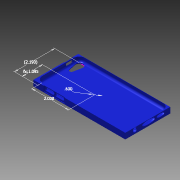
# Autodesk Inventor part: ipodcasev4
Saved by Autodesk Inventor 2014 SP2 (Build 180246200, 246)
## iProperties
Created: 2013-11-12
Part Number: ipodcasev4
Material: Generic
Document SubType Name: Modeling
Designer: jared.hale
Density: 1 g/cm^3
Appearance: Blue - Wall Paint - Glossy
Author: jared.hale
Autodesk Inventor part; units mm, degrees
ref_plane "YZ Plane" through (0, 0, 0) normal (1, 0, 0) x (0, 1, 0)
ref_plane "XZ Plane" through (0, 0, 0) normal (0, 1, 0) x (-1, 0, 0)
ref_plane "XY Plane" through (0, 0, 0) normal (0, 0, 1) x (1, 0, 0)
sketch "Sketch1" plane through (0, 0, 0) normal (0, 1, 0) x (-1, 0, 0)
  line L0 (-133.35, 69.85) -> (0, 69.85)
  line L1 (0, 69.85) -> (0, 0)
  line L2 (0, 0) -> (-133.35, 0)
  line L3 (-133.35, 0) -> (-133.35, 69.85)
  dimension "d0" = 133.35
  dimension "d2" = 69.85
  constraints: 8 end point, 2 parallel, 1 horizontal, 1 perpendicular
  measures "d0" distance between parallel lines of L1 L3
  measures "d2" distance between parallel lines of L2 L0
extrude "Extrusion1" add sketch "Sketch1" along normal blind 25.4
sketch "Sketch2" plane through (0, 25.4, 0) normal (0, 1, 0) x (1, 0, 0)
  line L0 (0, 0) -> (0, -69.85) projected
  line L1 (133.35, 0) -> (0, 0) projected
  line L2 (12.7, -5.08) -> (121.285, -5.08)
  line L3 (128.905, -12.7) -> (128.905, -56.388)
  line L4 (121.285, -64.008) -> (12.7, -64.008)
  line L5 (5.08, -56.388) -> (5.08, -12.7)
  arc A0 (12.7, -5.08) -> (5.08, -12.7) centre (12.7, -12.7) ccw
  arc A1 (5.08, -56.388) -> (12.7, -64.008) centre (12.7, -56.388) ccw
  arc A2 (121.285, -64.008) -> (128.905, -56.388) centre (121.285, -56.388) ccw
  arc A3 (128.905, -12.7) -> (121.285, -5.08) centre (121.285, -12.7) ccw
  dimension "d5" = 58.928
  dimension "d7" = 123.825
  dimension "d8" = 5.08
  dimension "d9" = 5.08
  dimension "d10" = 7.62
  constraints: 8 end point, 8 point on circle, 8 tangent, 4 centre point, 3 equal radius, 2 parallel, 1 horizontal, 1 perpendicular
  measures "d5" distance between parallel lines of L4 L2
  measures "d7" distance between parallel lines of L3 L5
  measures "d8" distance between parallel lines of L2 L1
  measures "d9" distance between parallel lines of L0 L5
  measures "d10" radius of A0
extrude "Extrusion2" cut sketch "Sketch2" against normal blind 6.4008
fillet "Fillet1" radius 3.175 8 edges at (126.6732, 18.9992, 7.3118) (128.905, 18.9992, 34.544) (126.6732, 18.9992, 61.7762) (66.9925, 18.9992, 64.008) (7.3118, 18.9992, 61.7762) (5.08, 18.9992, 34.544) (7.3118, 18.9992, 7.3118) (66.9925, 18.9992, 5.08)
sketch "Sketch3" plane through (5.08, 25.4, 56.388) normal (1, 0, 0) x (0, 0, -1)
  line L0 (43.688, 0) -> (43.688, -3.2258) projected
  line L1 (0, 0) -> (43.688, 0) projected
  line L2 (34.163, -1.397) -> (41.402, -1.397)
  line L3 (42.672, -2.667) -> (42.672, -3.175)
  line L4 (41.402, -4.445) -> (34.163, -4.445)
  line L5 (32.893, -3.175) -> (32.893, -2.667)
  arc A0 (42.672, -2.667) -> (41.402, -1.397) centre (41.402, -2.667) ccw
  arc A1 (41.402, -4.445) -> (42.672, -3.175) centre (41.402, -3.175) ccw
  arc A2 (32.893, -3.175) -> (34.163, -4.445) centre (34.163, -3.175) ccw
  arc A3 (34.163, -1.397) -> (32.893, -2.667) centre (34.163, -2.667) ccw
  point P0 (56.388, -25.4)
  dimension "d14" = 1.016
  dimension "d15" = 9.779
  dimension "d16" = 1.397
  dimension "d17" = 3.048
  dimension "d18" = 1.27
  constraints: 8 end point, 8 point on circle, 8 tangent, 4 centre point, 3 equal radius, 2 parallel, 1 horizontal, 1 perpendicular
  measures "d14" distance between parallel lines of L3 L0
  measures "d15" distance between parallel lines of L5 L3
  measures "d16" distance between parallel lines of L2 L1
  measures "d17" distance between parallel lines of L4 L2
  measures "d18" radius of A0
extrude "Extrusion3" cut sketch "Sketch3" along normal mid plane 50.8
sketch "Sketch4" plane through (121.285, 25.4, 64.008) normal (0, 0, -1) x (-1, 0, 0)
  line L0 (0, 0) -> (108.585, 0) projected
  line L1 (77.851, -4.953) -> (100.711, -4.953)
  line L2 (101.981, -3.683) -> (101.981, -2.54)
  line L3 (100.711, -1.27) -> (77.851, -1.27)
  line L4 (76.581, -2.54) -> (76.581, -3.683)
  arc A0 (101.981, -2.54) -> (100.711, -1.27) centre (100.711, -2.54) ccw
  arc A1 (100.711, -4.953) -> (101.981, -3.683) centre (100.711, -3.683) ccw
  arc A2 (77.851, -1.27) -> (76.581, -2.54) centre (77.851, -2.54) ccw
  arc A3 (76.581, -3.683) -> (77.851, -4.953) centre (77.851, -3.683) ccw
  point P0 (108.585, -3.2258)
  point P1 (121.285, -25.4)
  point P2 (116.205, -3.2258)
  dimension "d37" = 7.62
  dimension "d38" = 14.224
  dimension "d39" = 25.4
  dimension "d40" = 3.683
  dimension "d41" = 3.2258
  dimension "d42" = 1.27
  dimension "d43" = 1.27
  constraints: 8 end point, 8 point on circle, 8 tangent, 4 centre point, 3 equal radius, 2 parallel, 1 horizontal, 1 perpendicular
  measures "d37" distance of point (108.585, -3.226) point (116.205, -3.226)
  measures "d38" distance from line of point (116.205, -3.226) L2
  measures "d39" distance between parallel lines of L4 L2
  measures "d40" distance between parallel lines of L1 L3
  measures "d41" distance from line of point (116.205, -3.226) L0
  measures "d42" distance between parallel lines of L3 L0
  measures "d43" radius of A0
sketch "Sketch5" plane through (128.905, 25.4, 12.7) normal (-1, 0, 0) x (0, 0, 1)
  line L0 (43.688, -3.2258) -> (0, -3.2258) projected
  line L1 (0, 0) -> (43.688, 0) projected
  ellipse E0 centre (21.7805, -3.175) end of major axis (30.6705, -3.175) minor radius 2.54
  point P0 (-12.7, -25.4)
  dimension "d21" = 8.89
  dimension "d23" = 2.54
  dimension "d26" = 3.175
  constraints: 1 horizontal, 2 other
  measures "d26" distance from line of point (21.78, -3.175) L1
extrude "Extrusion4" cut sketch "Sketch5" along normal mid plane 50.8
sketch "Sketch6" plane through (128.905, 25.4, 12.7) normal (-1, 0, 0) x (0, 0, 1)
  ellipse E0 centre (21.7805, -3.175) end of major axis (12.8905, -3.175) minor radius 2.54 (30.6687, -3.2258) -> (12.8923, -3.2258) ccw projected
  line L0 (12.8923, -3.2258) -> (0, -3.2258) projected
  circle A0 centre (40.7035, -3.175) radius 2.794
  ellipse E1 centre (5.2705, -3.175) end of major axis (10.668, -3.175) minor radius 1.905
  point P0 (-12.7, -25.4)
  dimension "d35" = 5.3975
  dimension "d36" = 1.905
  dimension "d29" = 5.588
  dimension "d31" = 18.923
  dimension "d34" = 16.51
  constraints: 1 centre point, 1 horizontal, 3 other
  measures "d29" diameter of A0
  measures "d31" distance of point (21.78, -3.175) A0.centre
  measures "d34" distance of point (5.27, -3.175) point (21.78, -3.175)
extrude "Extrusion5" cut sketch "Sketch6" along normal mid plane 10.16
extrude "Extrusion6" cut sketch "Sketch4" along normal mid plane 50.8
sketch "Sketch7" plane through (0, 18.9992, 0) normal (0, 1, 0) x (1, 0, 0)
  line L0 (12.7, -8.255) -> (121.285, -8.255) projected
  line L1 (8.255, -56.388) -> (8.255, -12.7) projected
  arc A0 (16.7866, -12.9365) -> (7.3434, -12.9365) centre (12.065, -11.938) ccw
  arc A1 (9.58, -23.5125) -> (14.55, -23.5125) centre (12.065, -22.987) ccw
  line L2 (7.3434, -12.9365) -> (9.58, -23.5125)
  line L3 (16.7866, -12.9365) -> (14.55, -23.5125)
  point P0 (0, 0)
  point P1 (5.08, -5.08)
  dimension "d46" = 11.049
  dimension "d48" = 0
  dimension "d49" = 9.652
  dimension "d50" = 5.08
  dimension "d51" = 3.175
  dimension "d52" = 3.175
  dimension "d53" = 6.858
  dimension "d54" = 6.985
  constraints: 4 end point, 4 point on circle, 4 tangent, 2 centre point
  measures "d46" distance of A1.centre A0.centre
  measures "d48" horizontal distance of A0.centre A1.centre
  measures "d49" diameter of A0
  measures "d50" diameter of A1
  measures "d51" distance from line of point (5.08, -5.08) L0
  measures "d52" distance from line of point (5.08, -5.08) L1
  measures "d53" vertical distance of A0.centre point (5.08, -5.08)
  measures "d54" horizontal distance of A0.centre point (5.08, -5.08)
extrude "Extrusion7" cut sketch "Sketch7" along normal mid plane 50.8
ref_plane "Work Plane1" through (0, 0, 34.925) normal (0, 0, 1) x (1, 0, 0)
fillet "Fillet2" [suppressed]
sketch "Sketch10" plane through (0, 0, 34.925) normal (0, 0, 1) x (1, 0, 0)
  line L0 (15.1836, 18.9992) -> (121.285, 18.9992) projected
  line L1 (5.08, 24.13) -> (5.7032, 25.2095) projected
  line L2 (128.905, 24.13) -> (128.2818, 25.2095) projected
  line L3 (3.556, 25.8521) -> (3.556, 17.4752)
  line L4 (3.556, 17.4752) -> (130.429, 17.4752)
  line L5 (130.429, 17.4752) -> (130.429, 25.8521)
  line L6 (3.556, 25.8521) -> (-3.1756, 25.6598)
  line L7 (-3.1756, 25.6598) -> (-4.2851, -9.2303)
  line L8 (-4.2851, -9.2303) -> (140.2506, -12.8123)
  line L9 (140.2506, -12.8123) -> (141.3589, 31.9078)
  line L10 (141.3589, 31.9078) -> (130.429, 25.8521)
  point P0 (0, 0)
  dimension "d62" = 1.524
  dimension "d63" = 1.524
  dimension "d65" = 1.524
  constraints: 16 end point, 1 parallel, 1 perpendicular
  measures "d62" distance from line of L3 L1.start
  measures "d63" distance from line of L5 L2.start
  measures "d65" distance between parallel lines of L4 L0
extrude "Extrusion8" cut sketch "Sketch10" along normal mid plane 127
ref_plane "Work Plane2" through (66.9925, 22.1742, 43.3687) normal (-1, 0, 0) x (0, 0, 1)
sketch "Sketch11" plane through (66.9925, 22.1742, 43.3687) normal (-1, 0, 0) x (0, 0, 1)
  arc A0 (-38.2887, 0) -> (-35.1137, -3.175) centre (-35.1137, 0) ccw projected
  line L0 (-38.2887, 3.2258) -> (-38.2887, 0) projected
  line L1 (-37.019, 1.9558) -> (-36.3957, 3.0353) projected
  line L2 (-35.1137, -3.175) -> (-30.6687, -3.175) projected
  line L3 (-30.6687, -3.175) -> (13.0193, -3.175) projected
  line L4 (21.909, 1.9558) -> (21.2858, 3.0353) projected
  line L5 (20.6393, 3.2258) -> (20.6393, 0) projected
  arc A1 (17.4643, -3.175) -> (20.6393, 0) centre (17.4643, 0) ccw projected
  line L6 (23.433, 3.4455) -> (23.433, -4.699)
  line L7 (23.433, -4.699) -> (-38.543, -4.699)
  line L8 (-38.543, -4.699) -> (-38.543, 3.4455)
  line L9 (-38.543, 3.4455) -> (-45.2909, 4.3376)
  line L10 (-45.2909, 4.3376) -> (-44.8539, -8.6551)
  line L11 (-44.8539, -8.6551) -> (36.1582, -8.6551)
  line L12 (36.1582, -8.6551) -> (31.3237, 8.6218)
  line L13 (31.3237, 8.6218) -> (23.433, 3.4455)
  point P0 (-43.3687, -22.1742)
  point P1 (9.795, -3.175)
  dimension "d68" = 1.524
  dimension "d69" = 1.524
  dimension "d70" = 1.524
  constraints: 16 end point, 1 parallel, 1 perpendicular, 2 other
  measures "d68" distance from line of L8 L1.start
  measures "d69" distance from line of L6 L4.start
  measures "d70" distance between parallel lines of L7 L3
extrude "Extrusion9" cut sketch "Sketch11" along normal mid plane 152.4
sketch "Sketch12" plane through (20.574, 24.13, 66.8017) normal (0, 0, 1) x (1, 0, 0)
  line L0 (22.86, 0) -> (0, 0) projected
  line L1 (-16.764, 1.27) -> (-16.764, -3.4798) projected
  line L2 (10.4775, 0) -> (10.4775, -3.683)
  line L3 (10.4775, -3.683) -> (12.3825, -3.683)
  line L4 (12.3825, -3.683) -> (12.3825, 0)
  line L5 (22.86, -3.683) -> (0, -3.683) projected
  point P0 (-20.574, -24.13)
  point P1 (-16.764, 0.635)
  point P2 (-1.27, -2.413)
  point P3 (24.13, -2.413)
  dimension "d82" = 1.905
  dimension "d85" = 0
  dimension "d91" = 25.4
  dimension "d92" = 11.7475
  constraints: 6 end point, 2 perpendicular, 2 point on line, 1 parallel
  measures "d82" distance between parallel lines of L4 L2
  measures "d85" distance between parallel lines of L5 L3
  measures "d91" distance of point (24.13, -2.413) point (-1.27, -2.413)
  measures "d92" distance from line of point (-1.27, -2.413) L2
extrude "Extrusion10" add sketch "Sketch12" against normal blind 2.54
fillet "Fillet10" radius 1.27 4 edges at (32.9565, 20.447, 65.5317) (32.9565, 24.13, 65.5317) (31.0515, 24.13, 65.5317) (31.0515, 20.447, 65.5317)
chamfer "Chamfer3" distance 0.762 angle 45 4 edges at (12.065, 17.4752, 7.112) (15.6683, 17.4752, 18.2245) (12.065, 17.4752, 25.527) (8.4617, 17.4752, 18.2245)
ref_plane "Work Plane3" through (13.716, 17.4752, 62.357) normal (0, -1, 0) x (1, 0, 0)
sketch "Sketch14" plane through (13.716, 17.4752, 62.357) normal (0, -1, 0) x (1, 0, 0)
  line L0 (113.538, -55.626) -> (-6.985, -55.626) projected
  line L1 (-6.985, 0) -> (113.538, 0) projected
  circle A0 centre (42.164, -27.813) radius 7.62
  line L2 (-8.636, -38.863) -> (-8.636, -5.969) projected
  point P0 (0.4971, -55.499)
  point P1 (106.553, -55.626)
  point P2 (106.553, 0)
  point P3 (0, 0)
  point P4 (-13.716, -62.357)
  point P5 (0.0679, -55.626)
  point P6 (-6.985, -55.626)
  dimension "d103" = 27.813
  dimension "d104" = 55.626
  dimension "d105" = 50.8
  dimension "d106" = 15.24
  constraints: 1 centre point, 1 other
  measures "d103" distance from line of A0.centre L1
  measures "d105" distance from line of A0.centre L2
  measures "d106" diameter of A0
sketch "Sketch17" plane through (0, 25.4, 0) normal (0, 1, 0) x (1, 0, 0)
  line L0 (3.556, -66.8017) -> (130.429, -66.8017) projected
  line L1 (3.556, -4.8257) -> (3.556, -66.8017) projected
  line L2 (5.08, -13.716) -> (3.556, -13.716) projected
  line L3 (3.556, -13.716) -> (5.08, -13.716) projected
  line L4 (5.08, -23.495) -> (3.556, -23.495) projected
  line L5 (5.08, -23.495) -> (3.556, -23.495) projected
  line L6 (4.318, -24.13) -> (4.318, -13.081)
  line L7 (45.72, -66.0397) -> (18.288, -66.0397)
  line L8 (4.318, -24.511) -> (4.318, -24.13)
  line L9 (4.318, -12.7) -> (4.318, -13.157)
  line L10 (4.318, -24.511) -> (3.556, -25.273)
  line L11 (4.318, -24.511) -> (5.471, -24.511) construction
  line L12 (4.318, -12.7) -> (3.7438, -12.1258)
  line L13 (4.318, -12.7) -> (5.2745, -12.7) construction
  line L14 (18.288, -66.0397) -> (17.526, -66.8017)
  line L15 (45.72, -66.0397) -> (46.482, -66.8017)
  arc A0 (12.7, -4.8257) -> (3.556, -13.9697) centre (12.7, -13.9697) ccw projected
  point P0 (3.556, -55.372)
  point P1 (13.716, -65.532)
  point P2 (120.269, -65.532)
  point P3 (3.556, -13.716)
  point P4 (0, 0)
  point P5 (44.704, -66.8017)
  point P6 (32.9565, -66.8017)
  point P7 (31.0515, -66.8017)
  point P8 (19.304, -66.8017)
  point P9 (3.6899, -12.0719)
  dimension "d115" = 0.762
  dimension "d119" = 135
  dimension "d120" = 135
  dimension "d121" = 0.762
  dimension "d122" = 1.016
  dimension "d123" = 1.016
  dimension "d125" = 1.016
  constraints: 20 end point, 3 horizontal, 3 perpendicular, 3 point on line, 2 collinear, 1 point on circle, 3 other
  measures "d115" distance between parallel lines of L6 L1
  measures "d119" angle of L10 L11
  measures "d120" angle of L13 L12
  measures "d122" horizontal distance of point (44.704, -66.802) L7.start
  measures "d123" horizontal distance of point (19.304, -66.802) L7.end
  measures "d125" distance from line of L4 L8.start
extrude "Extrusion13" cut sketch "Sketch17" against normal blind 7.0866 contours L14 L7 L15 L0 | A0 L2 L6 L4 L1 | A0 L12 L9 L6 L2 | L4 L6 L8 L10 L1
fillet "Fillet20" radius 0.5387 4 edges at (18.288, 21.8567, 66.0397) (45.72, 21.8567, 66.0397) (4.318, 21.8567, 12.7) (4.318, 21.8567, 24.511)
fillet "Fillet21" radius 0.254 3 edges at (3.556, 21.8567, 25.273) (17.526, 21.8567, 66.8017) (46.482, 21.8567, 66.8017)
chamfer "Chamfer5" distance 0.762 angle 45 8 edges at (4.318, 20.955, 18.6055) (4.318, 21.327, 23.123) (4.318, 22.479, 23.495) (4.318, 23.631, 23.123) (4.318, 24.003, 18.6055) (4.318, 23.631, 14.088) (4.318, 22.479, 13.716) (4.318, 21.327, 14.088)
fillet "Fillet22" radius 0.762 8 edges at (4.318, 22.479, 12.9541) (4.318, 20.7882, 13.5492) (4.318, 20.1931, 18.6055) (4.318, 20.7882, 23.6618) (4.318, 22.479, 24.2569) (4.318, 24.1698, 23.6618) (4.318, 24.7649, 18.6055) (4.318, 24.1698, 13.5492)
sketch "Sketch18" plane through (32.9565, 20.447, 62.992) normal (1, 0, 0) x (0, 0, -1)
  line L0 (-1.2697, 1.27) -> (-3.0477, 1.27) projected
  arc A0 (-0.9829, 1.27) -> (-0.5051, 0) centre (2.159, 1.7272) ccw projected
  line L1 (-0.5051, 0) -> (0, 0) projected
  line L2 (-1.2697, 2.413) -> (-1.2697, 1.27) projected
  line L3 (-1.016, 3.683) -> (0, 3.683) projected
  line L4 (-1.016, 3.683) -> (-1.016, 2.413) projected
  line L5 (-3.0477, 2.413) -> (-3.0477, 3.683) projected
  line L6 (-3.0477, 3.683) -> (-1.2697, 3.683) projected
  line L7 (-1.2697, 2.413) -> (-3.0477, 2.413) projected
  arc A1 (-0.9829, 1.27) -> (-0.5051, 0) centre (2.159, 1.7272) ccw
  line L8 (-1.016, 3.683) -> (-1.016, 2.413)
  line L9 (-1.016, 2.413) -> (-1.016, 1.27)
  arc A2 (-1.016, 1.8415) -> (-0.9829, 1.27) centre (2.2895, 1.7462) ccw
  line L10 (-1.016, 3.683) -> (0, 3.683)
  line L11 (0, 3.683) -> (0, 0)
  line L12 (0, 0) -> (-0.5051, 0)
  line L13 (-1.2697, 3.683) -> (-1.2697, 2.413) projected
  point P0 (62.992, -20.447)
  constraints: 10 end point, 4 collinear, 4 point on circle, 2 centre point, 1 midpoint, 1 point on line, 1 tangent, 1 vertical, 1 other
extrude "Extrusion14" cut sketch "Sketch18" against normal up to surface (1.905 mm away) contours A2 L9 L4 L3 L11 L1 A0
sketch "Sketch19" plane through (31.0515, 21.717, 66.0397) normal (-1, 0, 0) x (0, 0, 1)
  arc A0 (-0.7951, 0) -> (-0.762, 0.5715) centre (-4.0675, 0.4762) ccw projected
  line L0 (-0.762, 1.143) -> (-0.762, 0.5715) projected
  line L1 (-0.762, 2.159) -> (-0.635, 2.159)
  line L2 (-0.635, 2.159) -> (-0.635, -1.016)
  line L3 (-0.635, -1.016) -> (-2.3942, -1.016)
  arc A1 (-5.2067, -2.7178) -> (-2.0317, 0.4572) centre (-5.2067, 0.4572) ccw projected
  line L4 (-0.762, 2.413) -> (-0.762, 1.143) projected
  line L5 (-0.762, 2.159) -> (-0.762, 0.5715)
  arc A2 (-2.3942, -1.016) -> (-0.762, 0.5715) centre (-2.3068, 0.527) ccw
  point P0 (-66.0397, -21.717)
  point P1 (0, 2.413)
  point P2 (0, -1.27)
  dimension "d140" = 0.254
  dimension "d141" = 0.254
  dimension "d142" = 0.127
  constraints: 8 end point, 2 perpendicular, 2 point on circle, 1 centre point, 1 collinear, 1 parallel, 1 tangent, 2 other
  measures "d140" distance from line of L3 point (0, -1.27)
  measures "d141" distance from line of point (0, 2.413) L1
  measures "d142" distance between parallel lines of L4 L2
extrude "Extrusion15" [suppressed]
fillet "Fillet23" [suppressed]
fillet "Fillet24" radius 0.3175 5 edges at (130.429, 20.32, 17.9689) (130.429, 24.13, 17.9721) (130.429, 19.685, 34.4785) (130.429, 24.765, 34.4823) (130.429, 22.225, 50.6095)
chamfer "Chamfer6" distance 0.381 angle 45 16 edges at (31.0515, 22.2885, 66.0397) (30.6795, 23.758, 66.0397) (25.1778, 24.13, 66.0397) (19.676, 23.758, 66.0397) (19.304, 22.2885, 66.0397) (19.676, 20.819, 66.0397) (25.1778, 20.447, 66.0397) (30.6795, 20.819, 66.0397) (32.9565, 22.2885, 66.0397) (33.3285, 20.819, 66.0397) (38.8302, 20.447, 66.0397) (44.332, 20.819, 66.0397) (44.704, 22.2885, 66.0397) (44.332, 23.758, 66.0397) (38.8302, 24.13, 66.0397) (33.3285, 23.758, 66.0397)
fillet "Fillet25" radius 0.635 16 edges at (31.4325, 22.2885, 66.0397) (30.9489, 24.0274, 66.0397) (25.1778, 24.511, 66.0397) (19.4066, 24.0274, 66.0397) (18.923, 22.2885, 66.0397) (19.4066, 20.5496, 66.0397) (25.1778, 20.066, 66.0397) (30.9489, 20.5496, 66.0397) (38.8302, 20.066, 66.0397) (44.6014, 20.5496, 66.0397) (45.085, 22.2885, 66.0397) (44.6014, 24.0274, 66.0397) (38.8303, 24.511, 66.0397) (33.0591, 24.0274, 66.0397) (32.5755, 22.2885, 66.0397) (33.0591, 20.5496, 66.0397)
fillet "Fillet26" [suppressed]
fillet "Fillet27" [suppressed]
equation "\"d92\" = -0.5 * d82 + 0.5 * d91"
equation "\"d103\" = 0.5 * d104"
body "Solid1"
